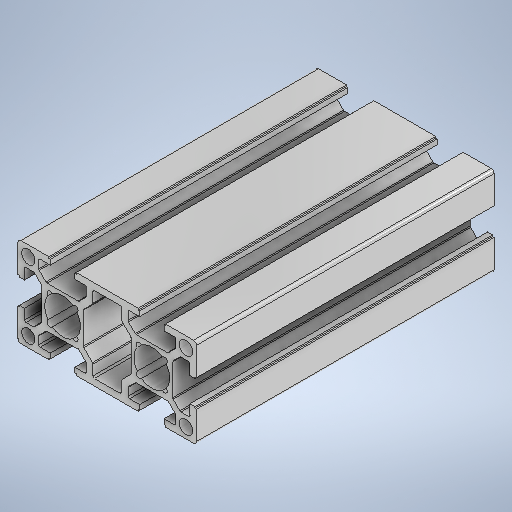
# Autodesk Inventor part: Perfil 30×60 6 rasgos_001
Saved by Autodesk Inventor 2026 (Build 300175000, 175)
## iProperties
Created: 2025-04-04
Part Number: Perfil 30×60 6 rasgos_001
Material: Aluminum 6061
Document SubType Name: Modeling
Designer: Carlos Dias
Density: 2.7 g/cm^3
Appearance: Aluminum - Polished
Author: Carlos Dias
Autodesk Inventor part; units mm, degrees
sketch "Sketch1" plane through (0, 0, 0) normal (0, 0, 1) x (1, 0, 0)
  line L0 (-30, 15) -> (-30, 0) construction
  line L1 (-30, 15) -> (-30, 4.1) construction
  line L2 (-30, 4.1) -> (-27.8, 4.1) construction
  line L3 (-27.8, 8) -> (-27.8, 4.1) construction
  line L4 (-30, 4.1) -> (-29.5, 4.1) construction
  line L5 (-29.5, 4.1) -> (-29.5, 4.6)
  line L6 (-29.5, 4.6) -> (-30, 4.6)
  line L7 (-30, 4.6) -> (-30, 4.1) construction
  line L8 (-30, 15) -> (-30, 4.6) construction
  line L9 (-27.8, 4.1) -> (-29.5, 4.1)
  line L10 (-30, 15) -> (0, 15) construction
  arc A0 (-29, 15) -> (-30, 14) centre (-29, 14) ccw
  line L11 (-30, 14) -> (-30, 4.6)
  circle A1 centre (-26.5, 11.5) radius 2.25
  circle A2 centre (-15, 0) radius 6 construction
  line L12 (-19.1, 15) -> (-19.1, 12.8) construction
  line L13 (-19.1, 15) -> (-19.6, 15) construction
  line L14 (-19.6, 15) -> (-19.6, 14.5)
  line L15 (-19.6, 14.5) -> (-19.1, 14.5)
  line L16 (-19.1, 14.5) -> (-19.1, 15) construction
  line L17 (-19.1, 14.5) -> (-19.1, 12.8)
  line L18 (-29, 15) -> (-19.6, 15)
  line L19 (-23, 12.8) -> (-19.1, 12.8) construction
  line L20 (-27.8, 8) -> (-22, 8) construction
  arc A3 (-27.3, 8) -> (-27.8, 7.5) centre (-27.3, 7.5) ccw
  line L21 (-27.8, 7.5) -> (-27.8, 4.1)
  line L22 (-22, 5.4444) -> (-22, 0) construction
  line L23 (-30, 15) -> (-15, 0) construction
  circle A4 centre (-19.2426, 4.2426) radius 1 construction
  circle A5 centre (-15, 0) radius 6 construction
  circle A6 centre (-19.2426, -4.2426) radius 1 construction
  circle A7 centre (-15, 0) radius 6 construction
  circle A8 centre (-10.7574, -4.2426) radius 1 construction
  circle A9 centre (-15, 0) radius 6 construction
  circle A10 centre (-10.7574, 4.2426) radius 1 construction
  line L24 (-20.4444, 7) -> (-15, 7) construction
  line L25 (-23, 9.5556) -> (-20.4444, 7) construction
  line L26 (-24.5556, 8) -> (-22, 5.4444) construction
  line L27 (-23, 12.8) -> (-23, 9.5556) construction
  line L28 (-15, 7) -> (-9.5556, 7) construction
  line L29 (-10.9, 12.8) -> (-7, 12.8) construction
  line L30 (-10.9, 15) -> (-10.9, 12.8) construction
  line L31 (-10.9, 15) -> (-10.4, 15) construction
  line L32 (-10.4, 15) -> (-10.4, 14.5)
  line L33 (-10.4, 14.5) -> (-10.9, 14.5)
  line L34 (-10.9, 14.5) -> (-10.9, 15) construction
  line L35 (-10.9, 14.5) -> (-10.9, 12.8)
  line L36 (-7, 12.8) -> (-7, 9.5556) construction
  line L37 (-7, 9.5556) -> (-9.5556, 7) construction
  line L38 (-8, 5.4444) -> (-8, 0) construction
  line L39 (-4.8, 8.6444) -> (-8, 5.4444) construction
  line L40 (-4.8, 12.8) -> (-4.8, 8.6444) construction
  arc A11 (-19.8884, 3.4791) -> (-21, 0) centre (-15, 0) ccw
  arc A12 (-11.5209, 4.8884) -> (-18.4791, 4.8884) centre (-15, 0) ccw
  arc A13 (-9, 0) -> (-10.1116, 3.4791) centre (-15, 0) ccw
  arc A14 (-18.4791, 4.8884) -> (-19.8884, 3.4791) centre (-19.2426, 4.2426) ccw
  arc A15 (-10.1116, 3.4791) -> (-11.5209, 4.8884) centre (-10.7574, 4.2426) ccw
  line L41 (-36.2485, 0) -> (6.0414, 0) projected
  line L42 (0, 15) -> (0, 15) construction
  arc A16 (-24.4092, 7.8536) -> (-24.7627, 8) centre (-24.7627, 7.5) ccw
  arc A17 (-22, 5.2373) -> (-22.1464, 5.5908) centre (-22.5, 5.2373) ccw
  line L43 (-27.3, 8) -> (-24.7627, 8)
  line L44 (-24.4092, 7.8536) -> (-22.1464, 5.5908)
  line L45 (-22, 5.2373) -> (-22, 0)
  line L46 (-22, 0) -> (-21, 0)
  arc A18 (-23, 9.7627) -> (-22.8536, 9.4092) centre (-22.5, 9.7627) ccw
  arc A19 (-20.5908, 7.1464) -> (-20.2373, 7) centre (-20.2373, 7.5) ccw
  arc A20 (-22.5, 12.8) -> (-23, 12.3) centre (-22.5, 12.3) ccw
  arc A21 (-7, 12.3) -> (-7.5, 12.8) centre (-7.5, 12.3) ccw
  arc A22 (-7.1464, 9.4092) -> (-7, 9.7627) centre (-7.5, 9.7627) ccw
  arc A23 (-9.7627, 7) -> (-9.4092, 7.1464) centre (-9.7627, 7.5) ccw
  arc A24 (-7.8536, 5.5908) -> (-8, 5.2373) centre (-7.5, 5.2373) ccw
  arc A25 (-4.9464, 8.4979) -> (-4.8, 8.8515) centre (-5.3, 8.8515) ccw
  arc A26 (-4.3, 12.8) -> (-4.8, 12.3) centre (-4.3, 12.3) ccw
  line L47 (-8, 5.2373) -> (-8, 0)
  line L48 (-8, 0) -> (-9, 0)
  line L49 (-4.9464, 8.4979) -> (-7.8536, 5.5908)
  line L50 (-4.8, 12.3) -> (-4.8, 8.8515)
  line L51 (-22.5, 12.8) -> (-19.1, 12.8)
  line L52 (-23, 12.3) -> (-23, 9.7627)
  line L53 (-22.8536, 9.4092) -> (-20.5908, 7.1464)
  line L54 (-20.2373, 7) -> (-9.7627, 7)
  line L55 (-7.1464, 9.4092) -> (-9.4092, 7.1464)
  line L56 (-7, 12.3) -> (-7, 9.7627)
  line L57 (-10.9, 12.8) -> (-7.5, 12.8)
  line L58 (-4.3, 12.8) -> (0, 12.8)
  line L59 (-10.4, 15) -> (0, 15)
  line L60 (0, 15) -> (0, 12.8)
  point P0 (0, 0)
  dimension "d33" = 12
  dimension "d2" = 15
  dimension "d3" = 4.1
  dimension "d4" = 2.2
  dimension "d6" = 0.5
  dimension "d7" = 1
  dimension "d8" = 4.5
  dimension "d32" = 15
  dimension "d34" = 4.1
  dimension "d37" = 26.5
  dimension "d38" = 11.5
  dimension "d39" = 1.25
  dimension "d40" = 0.5
  dimension "d42" = 8
  dimension "d46" = 2
  dimension "d49" = 360
  dimension "d51" = 1
  dimension "d52" = 1.1
  dimension "d54" = 8.2
  dimension "d56" = 2.2
  dimension "d57" = 1
  dimension "d58" = 2.2
  dimension "d75" = 2.2
  dimension "d76" = 4.3
  dimension "d77" = 30
  constraints: 120 end point, 40 point on circle, 32 point on line, 25 tangent, 23 centre point, 19 vertical, 18 horizontal, 11 equal radius, 10 coincident, 10 equal length, 9 parallel, 8 horizontal alignment, 7 vertical alignment, 3 perpendicular, 2 concentric, 1 midpoint, 41 other
  measures "d2" distance of L0.start L0.end
  measures "d3" vertical distance of point (0, 0) L1.end
  measures "d4" distance of L1.end L2.end
  measures "d6" distance of L5.end L6.end
  measures "d7" radius of A0
  measures "d8" diameter of A1
  measures "d32" distance of point (0, 0) point (-15, 0)
  measures "d34" horizontal distance of L12.start point (-15, 0)
  measures "d37" horizontal distance of point (0, 0) A1.centre
  measures "d38" vertical distance of point (0, 0) A1.centre
  measures "d39" distance edge to line of A1 L20
  measures "d40" radius of A3
  measures "d42" horizontal distance of L1.end L22.end
  measures "d46" diameter of A4
  measures "d52" distance between parallel lines of L23 L25
  measures "d54" distance of L29.start L12.end
  measures "d56" distance of L29.end L40.start
  measures "d58" distance between parallel lines of L37 L39
  measures "d75" distance between parallel lines of L10 L58
  measures "d76" distance of L58.start L58.end
  measures "d77" horizontal distance of point (0, 0) L0.start
extrude "Extrusion2" add sketch "Sketch1" along normal mid plane 100 contours L5 L6 L11 A0 L18 L14 L15 L17 L51 A20 L52 A18 L53 A19 L54 A23 L55 A22 L56 A21 L57 L35 L33 L32 L59 L60 L58 A26 L50 A25 L49 A24 L47 L41 A13 A15 A12 A14 A11 L45 A17 L44 A16 L43 A3 L21 L9
mirror "Mirror3" about plane through (0, 0, 0) normal (1, 0, 0) of "Extrusion2"
mirror "Mirror4" about plane through (0, 0, 0) normal (0, 1, 0) of "Extrusion2", "Mirror3"
equation "\"d52\" = 0.5 * d4"
equation "\"d56\" = d4"
equation "\"d57\" = d51"
equation "\"d58\" = d4"
body "Solid2"
